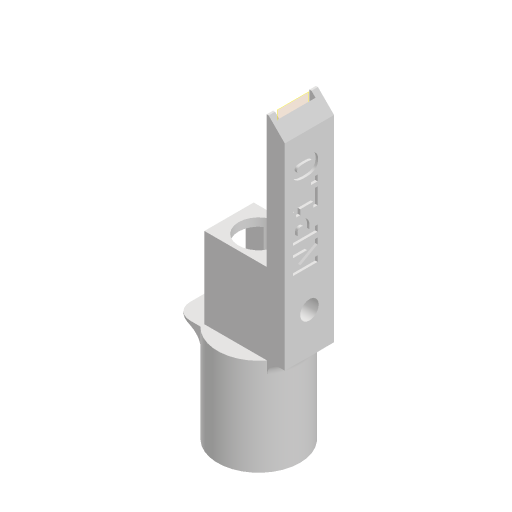
# Autodesk Inventor part: surgical_holder
Saved by Autodesk Inventor 2023 (Build 270158000, 158)
## iProperties
Created: 2023-01-31
Part Number: surgical_holder
Material: Generic
Document SubType Name: Modeling
Designer: mmelin
Density: 1 g/cm^3
Appearance: Default
Author: mmelin
Autodesk Inventor part; units mm, degrees
ref_plane "YZ Plane" through (0, 0, 0) normal (1, 0, 0) x (0, 1, 0)
ref_plane "XZ Plane" through (0, 0, 0) normal (0, 1, 0) x (-1, 0, 0)
ref_plane "XY Plane" through (0, 0, 0) normal (0, 0, 1) x (1, 0, 0)
ref_plane "Work Plane2" through (0.5918, -11.5934, -3.2844) normal (1, 0, 0) x (0, 0, -1)
sketch "Sketch2" plane through (0.5918, -11.5934, -3.2844) normal (1, 0, 0) x (0, 0, -1)
  line L0 (0.8156, 0) -> (0.8156, -11.35) projected
  line L1 (-3.2844, 0) -> (-3.2844, -15.35) projected
  line L2 (0.8156, 0) -> (-3.2844, 0) projected
  line L3 (1.8156, 0) -> (-4.2844, 0)
  line L4 (-4.2844, 0) -> (-4.2844, -11.35)
  line L5 (-4.2844, -11.35) -> (1.8156, -11.35)
  line L6 (1.8156, -11.35) -> (1.8156, 0)
  line L7 (0.8156, -11.35) -> (-2.0046, -11.35) projected
  point P0 (-3.2844, 11.5934)
  point P1 (0.8156, 0)
  point P2 (0.8156, -11.35)
  point P3 (-3.2844, -11.35)
  dimension "d81" = 1
  dimension "d82" = 1
  constraints: 8 end point, 2 collinear, 2 parallel, 1 horizontal, 1 perpendicular
  measures "d81" distance between parallel lines of L6 L0
  measures "d82" distance between parallel lines of L1 L4
extrude "arm_base" add sketch "Sketch2" along normal blind 1.5
sketch "Sketch22" plane through (0.5918, -11.5934, -3.2844) normal (-1, 0, 0) x (0, 0, 1)
  line L0 (4.2844, -11.35) -> (-1.8156, -11.35) projected
  line L1 (-1.8156, -11.35) -> (-1.0156, -11.35)
  line L2 (-1.0156, -11.35) -> (-1.0156, 0)
  line L3 (-1.0156, 0) -> (-1.8156, 0)
  line L4 (-1.8156, 0) -> (-1.8156, -11.35)
  line L5 (4.2844, -11.35) -> (-1.8156, -11.35) projected
  line L6 (4.2844, -11.35) -> (3.4844, -11.35)
  line L7 (3.4844, -11.35) -> (3.4844, 0)
  line L8 (3.4844, 0) -> (4.2844, 0)
  line L9 (4.2844, 0) -> (4.2844, -11.35)
  line L10 (-0.8156, 0) -> (-0.8156, -11.35) projected
  line L11 (3.2844, 0) -> (3.2844, -15.35) projected
  line L12 (-1.8156, 0) -> (4.2844, 0) projected
  point P0 (3.2844, 11.5934)
  point P1 (3.4844, -11.35)
  dimension "d83" = 0.2
  dimension "d84" = 0.2
  constraints: 16 end point, 4 parallel, 2 horizontal, 2 perpendicular, 1 collinear, 1 point on line
  measures "d83" distance between parallel lines of L10 L2
  measures "d84" distance between parallel lines of L11 L7
extrude "arm_tabs" add sketch "Sketch22" along normal blind 0.75 contours L0 L7 L8 L9 | L0 L4 L3 L2
sketch "Sketch23" plane through (2.0918, -22.9434, -5.1) normal (0, -1, 0) x (1, 0, 0)
  line L0 (-1.5, 0.8) -> (-2.25, 0.8) projected
  line L1 (-2.25, 0) -> (-2.25, 0.8) projected
  line L2 (-2.25, 5.3) -> (-2.25, 6.1) projected
  line L3 (-1.5, 5.3) -> (-2.25, 5.3) projected
  line L4 (-1.5, 5.3) -> (-1.5, 0.8) projected
  line L5 (0, 6.1) -> (0, 0) projected
  line L6 (-2.25, 6.1) -> (0, 6.1) projected
  line L7 (-1.5, 0.8) -> (-2.008, 0.8)
  line L8 (-2.008, 0.8) -> (-2.008, 3.8182)
  line L9 (-2.008, 3.8182) -> (-1.5, 3.8182)
  line L10 (-1.5, 3.8182) -> (-1.5, 0.8)
  line L11 (-2.25, 0) -> (0, 0) projected
  line L12 (-1.5, 0.8) -> (-2.25, 0.8) projected
  line L13 (-2.25, 0) -> (-2.25, 0.8) projected
  line L14 (-2.25, 5.3) -> (-2.25, 6.1) projected
  line L15 (-1.5, 5.3) -> (-2.25, 5.3) projected
  line L16 (-2.25, 0) -> (0, 0) projected
  line L17 (-2.008, 0.9187) -> (-2.008, 4.0182)
  line L18 (-2.9625, 4.0182) -> (-1.5, 4.0182) projected
  point P0 (-2.0918, 5.1)
  point P1 (0, 0)
  point P2 (-1.5, 5.2)
  point P3 (-1.5, 0.9)
  point P4 (-1.5, 3.8182)
  point P5 (0, 6.1)
  point P6 (-2.25, 6.1)
  dimension "d145" = 0.508
  dimension "d146" = 0.2
  constraints: 10 end point, 2 parallel, 2 perpendicular, 1 collinear, 1 horizontal, 1 point on line, 3 other
  measures "d145" distance between parallel lines of L17 L4
  measures "d146" distance between parallel lines of L18 L9
extrude "cut_out" add sketch "Sketch23" along normal blind 15 contours L4 L3 L2 L6 L5 L11 L1 L0 | L0 L8 L9 L4
chamfer "Chamfer1" distance 2 angle 45 1 edges at (2.0918, -11.5934, -2.05)
sketch "Sketch25" plane through (-0.1582, -11.5934, -3.2844) normal (-1, 0, 0) x (0, 0, 1)
  line L0 (0.0652, -16.35) -> (3.0834, -16.35)
  line L1 (4.2844, -26.35) -> (4.2844, -16.35)
  line L2 (4.2844, -16.35) -> (-1.8156, -16.35)
  line L3 (-1.8156, -16.35) -> (-1.8156, -26.35)
  line L4 (-1.8156, 0) -> (-1.8156, -26.35) projected
  line L5 (4.2844, 0) -> (4.2844, -26.35) projected
  line L6 (-1.8156, -26.35) -> (4.2844, -26.35)
  line L7 (4.2844, -26.35) -> (3.4844, -26.35) projected
  point P0 (3.2844, 11.5934)
  dimension "d131" = 10
  constraints: 10 end point, 4 collinear, 1 parallel
  measures "d131" distance between parallel lines of L2 L6
extrude "slider_box" add sketch "Sketch25" along normal blind 7.7
sketch "Sketch26" plane through (-7.8582, -11.5934, -3.2844) normal (-1, 0, 0) x (0, 0, 1)
  line L0 (-1.8156, -26.35) -> (4.2844, -26.35) projected
  line L1 (3.2844, -25.35) -> (-0.8156, -25.35)
  line L2 (-0.8156, -25.35) -> (-0.8156, -17.35)
  line L3 (-0.8156, -17.35) -> (3.2844, -17.35)
  line L4 (3.2844, -17.35) -> (3.2844, -25.35)
  line L5 (4.2844, -26.35) -> (4.2844, -16.35) projected
  line L6 (4.2844, -16.35) -> (-1.8156, -16.35) projected
  line L7 (-1.8156, -16.35) -> (-1.8156, -26.35) projected
  point P0 (3.2844, 11.5934)
  dimension "d97" = 1
  dimension "d147" = 1
  dimension "d148" = 1
  dimension "d149" = 1
  constraints: 8 end point, 2 parallel, 1 horizontal, 1 perpendicular
  measures "d97" distance between parallel lines of L0 L1
  measures "d147" distance between parallel lines of L5 L4
  measures "d148" distance between parallel lines of L6 L3
  measures "d149" distance between parallel lines of L7 L2
extrude "slider_cutout" cut sketch "Sketch26" against normal blind 7.7 contours L1 L2 L3 L4
sketch "Sketch27" plane through (2.0918, -37.9434, -5.1) normal (0, -1, 0) x (1, 0, 0)
  circle A0 centre (-6.2786, 3.05) radius 5.1
  line L0 (0.1377, 6.1) -> (-9.3123, 6.1)
  line L1 (0, 0) -> (-9.95, 0) projected
  line L2 (-6.2786, 3.05) -> (-6.2786, 0) construction
  line L3 (-6.2786, 3.05) -> (-6.2786, 6.1) construction
  line L4 (-11.0572, 5.1) -> (-11.0572, 1) projected
  line L5 (-1.5, 1) -> (-1.5, 5.1) projected
  line L6 (-6.2786, 3.05) -> (-11.0572, 3.05) construction
  line L7 (-6.2786, 3.05) -> (-1.5, 3.05) construction
  line L8 (0, 6.1) -> (-9.95, 6.1) projected
  point P0 (-2.0918, 5.1)
  point P1 (-9.95, 0)
  point P2 (-2.25, 0.019)
  dimension "d103" = 10.2
  constraints: 10 end point, 3 collinear, 2 midpoint, 2 point on line, 1 centre point, 1 vertical, 2 other
  measures "d103" diameter of A0
extrude "cylinder_post" add sketch "Sketch27" along normal blind 12
fillet "Fillet2" radius 1.8 1 edges at (-3.9788, -37.9434, -5.1)
sketch "Sketch28" plane through (-4.1868, -49.9434, -2.05) normal (0, -1, 0) x (1, 0, 0)
  circle A0 centre (0, 0) radius 5.1 projected
  circle A1 centre (0, 0) radius 4.1
  point P0 (4.1868, 2.05)
  dimension "d108" = 8.2
  constraints: 1 centre point, 1 coincident
  measures "d108" diameter of A1
extrude "post_cutout" cut sketch "Sketch28" against normal blind 9 contours A1
sketch "Sketch29" plane through (-4.1868, -40.9434, -2.05) normal (0, -1, 0) x (1, 0, 0)
  circle A0 centre (0, 0) radius 4.1 projected
  circle A1 centre (0, 0) radius 2.9
  point P0 (4.1868, 2.05)
  dimension "d111" = 5.8
  constraints: 1 centre point, 1 coincident
  measures "d111" diameter of A1
extrude "well" add sketch "Sketch29" along normal blind 8
fillet "Fillet4" radius 2 1 edges at (-0.0993, -37.0434, -5.1)
sketch "Sketch32" plane through (2.0918, -11.5934, -3.2844) normal (1, 0, 0) x (0, 0, -1)
  circle A0 centre (-1.2344, -21.35) radius 1.15
  line L0 (-1.2344, -21.35) -> (-1.2344, -25.35) construction
  line L1 (-1.2344, -21.35) -> (-1.2344, -17.35) construction
  line L2 (-1.2344, -21.35) -> (-3.2844, -21.35) construction
  line L3 (-1.2344, -21.35) -> (0.8156, -21.35) construction
  line L4 (-3.2844, -17.35) -> (-3.2844, -25.35) projected
  line L5 (0.8156, -17.35) -> (-3.2844, -17.35) projected
  line L6 (-3.2844, -25.35) -> (0.8156, -25.35) projected
  line L7 (0.8156, -25.35) -> (0.8156, -17.35) projected
  point P0 (-3.2844, 11.5934)
  dimension "d122" = 2.3
  constraints: 8 end point, 4 midpoint, 3 collinear, 2 perpendicular, 1 centre point, 1 point on line, 1 vertical
  measures "d122" diameter of A0
sketch "Sketch33" plane through (2.0918, -37.9434, -5.1) normal (0, 1, 0) x (1, 0, 0)
  arc A0 (-9.95, 0.4899) -> (-2.1911, -6.1) centre (-6.2786, -3.05) ccw projected
  line L0 (-9.95, -6.5899) -> (-13.23, -6.5899)
  line L1 (-13.23, -6.5899) -> (-13.23, 0.4899)
  line L2 (-13.23, 0.4899) -> (-9.95, 0.4899)
  line L3 (-9.95, 0.4899) -> (-9.95, -6.5899)
  point P0 (-2.0918, -5.1)
  point P1 (-1.6215, -0.9)
  point P2 (-1.5, -4.8319)
  point P3 (-9.4673, -7.0302)
  point P4 (-9.45, 0.918)
  point P5 (-9.45, -7.044)
  point P6 (-9.45, 0.918)
  dimension "d137" = 3.28
  constraints: 8 end point, 2 parallel, 1 horizontal, 1 perpendicular, 1 point on circle
  measures "d137" distance of L0.start L0.end
extrude "side_tab" add sketch "Sketch33" against normal blind 0.2
fillet "Fillet5" radius 2 1 edges at (-9.2868, -38.1434, -2.05)
fillet "Fillet6" radius 2 2 edges at (-11.1382, -38.0434, 1.4899) (-11.1382, -38.0434, -5.5899)
sketch "Sketch36" plane through (-0.1582, -27.9434, 0.2) normal (0, 1, 0) x (1, 0, 0)
  line L0 (0.75, 1.4818) -> (0.242, 1.4818) projected
  line L1 (0.242, 1.4818) -> (0.75, 1.4818)
  line L2 (0.75, 1.4818) -> (0.75, 0)
  line L3 (0.75, 0) -> (0.242, 0)
  line L4 (0.242, 0) -> (0.242, 1.4818)
  line L5 (0, 0) -> (0, 4.5) projected
  line L6 (0.242, 1.4818) -> (0.242, 4.5) projected
  line L7 (0, 4.5) -> (0.242, 4.5)
  line L8 (0, 0) -> (0, -0.8) projected
  line L9 (0, 0) -> (0.242, 0)
  point P0 (0.1582, 0.2)
  point P1 (0.75, 1.4818)
  point P2 (0, -0.9)
  constraints: 12 end point, 2 parallel, 2 perpendicular, 1 horizontal
extrude "fill_gaps" add sketch "Sketch36" against normal up to surface (10 mm away)
extrude "screw_hole" cut sketch "Sketch32" against normal up to surface (2.25 mm away) contours A0
fillet "Fillet7" radius 1.5 2 edges at (0.6535, -37.9434, -0.4432) (0.5192, -37.9434, -4.0156)
sketch "Sketch37" plane through (-4.1868, -40.9434, -2.05) normal (0, -1, 0) x (1, 0, 0)
  circle A0 centre (0, 0) radius 4.1 projected
  circle A1 centre (0, 0) radius 1.5
  point P0 (4.1868, 2.05)
  dimension "d138" = 3
  constraints: 1 centre point, 1 coincident
  measures "d138" diameter of A1
extrude "screw_hole_2" cut sketch "Sketch37" against normal up to surface (13 mm away) contours A1
sketch "Sketch38" plane through (-0.1582, -27.9434, 1) normal (0, 1, 0) x (-1, 0, 0)
  circle A0 centre (4.0286, -3.05) radius 1.5 projected
  circle A1 centre (4.0286, -3.05) radius 2.5
  point P0 (-0.1582, -1)
  dimension "d141" = 5
  constraints: 1 centre point, 1 coincident
  measures "d141" diameter of A1
extrude "screw_hole_3" cut sketch "Sketch38" against normal blind 11
sketch "Sketch39" plane through (2.0918, -11.5934, -3.2844) normal (1, 0, 0) x (0, 0, -1)
  line L0 (-3.3432, -17.034) -> (-3.3432, -3.22) construction
  line L1 (-3.3432, -3.22) -> (1.1831, -3.22) construction
  line L2 (1.1831, -3.22) -> (1.1831, -17.034) construction
  line L3 (1.1831, -17.034) -> (-3.3432, -17.034) construction
  line L4 (-0.2314, -14.1052) -> (-0.2314, -14.8417)
  line L5 (-0.2314, -14.8417) -> (-2.357, -16.0182)
  line L6 (-2.357, -16.0182) -> (-0.2314, -16.0182)
  line L7 (-0.2314, -16.0182) -> (-0.2314, -16.7177)
  line L8 (-0.2314, -16.7177) -> (-3.2814, -16.7177)
  line L9 (-3.2814, -16.7177) -> (-3.2814, -15.7785)
  line L10 (-3.2814, -15.7785) -> (-1.5339, -14.8046)
  line L11 (-1.5339, -14.8046) -> (-3.2814, -14.8046)
  line L12 (-3.2814, -14.8046) -> (-3.2814, -14.1052)
  line L13 (-3.2814, -14.1052) -> (-0.2314, -14.1052)
  spline S0 degree 2 poles (-2.3199, -11.1392) (-2.1074, -11.1392) (-1.7218, -11.2751) (-1.5933, -11.4012) knots 0 0 0 1 2 2 2
  spline S1 degree 2 poles (-1.5933, -11.4012) (-1.5117, -11.4778) (-1.3782, -11.6657) (-1.3313, -11.7769) knots 0 0 0 1 2 2 2
  spline S2 degree 2 poles (-1.3313, -11.7769) (-1.2843, -11.8906) (-1.2299, -12.155) (-1.2299, -12.3182) knots 0 0 0 1 2 2 2
  line L14 (-1.2299, -12.3182) -> (-1.2299, -12.7186)
  line L15 (-1.2299, -12.7186) -> (-0.2314, -12.7186)
  line L16 (-0.2314, -12.7186) -> (-0.2314, -13.4848)
  line L17 (-0.2314, -13.4848) -> (-3.2814, -13.4848)
  line L18 (-3.2814, -13.4848) -> (-3.2814, -12.3009)
  spline S3 degree 2 poles (-3.2814, -12.3009) (-3.2814, -12.0389) (-3.185, -11.6558) (-3.0812, -11.5001) knots 0 0 0 1 2 2 2
  spline S4 degree 2 poles (-3.0812, -11.5001) (-2.965, -11.327) (-2.5844, -11.1392) (-2.3199, -11.1392) knots 0 0 0 1 2 2 2
  spline S5 degree 2 poles (-2.3001, -11.9252) (-2.4311, -11.9252) (-2.6165, -12.0488) (-2.6511, -12.1328) knots 0 0 0 1 2 2 2
  spline S6 degree 2 poles (-2.6511, -12.1328) (-2.6981, -12.2415) (-2.7129, -12.4393) (-2.7129, -12.6098) knots 0 0 0 1 2 2 2
  line L19 (-2.7129, -12.6098) -> (-2.7129, -12.7186)
  line L20 (-2.7129, -12.7186) -> (-1.7984, -12.7186)
  line L21 (-1.7984, -12.7186) -> (-1.7984, -12.6642)
  spline S7 degree 2 poles (-1.7984, -12.6642) (-1.7984, -12.5579) (-1.8033, -12.3651) (-1.8157, -12.2935) knots 0 0 0 1 2 2 2
  spline S8 degree 2 poles (-1.8157, -12.2935) (-1.8256, -12.2317) (-1.8849, -12.0957) (-1.922, -12.0586) knots 0 0 0 1 2 2 2
  spline S9 degree 2 poles (-1.922, -12.0586) (-1.9961, -11.9796) (-2.1617, -11.9252) (-2.3001, -11.9252) knots 0 0 0 1 2 2 2
  line L22 (-0.2314, -8.6305) -> (-0.2314, -10.6449)
  line L23 (-0.2314, -10.6449) -> (-0.7628, -10.6449)
  line L24 (-0.7628, -10.6449) -> (-0.7628, -10.0022)
  line L25 (-0.7628, -10.0022) -> (-2.3768, -10.0022)
  line L26 (-2.3768, -10.0022) -> (-2.3768, -10.6449)
  line L27 (-2.3768, -10.6449) -> (-2.8736, -10.6449)
  spline S10 degree 2 poles (-2.8736, -10.6449) (-2.8736, -10.504) (-2.9106, -10.2247) (-2.9502, -10.1407) knots 0 0 0 1 2 2 2
  spline S11 degree 2 poles (-2.9502, -10.1407) (-2.9996, -10.0443) (-3.1652, -9.9355) (-3.2888, -9.9256) knots 0 0 0 1 2 2 2
  line L28 (-3.2888, -9.9256) -> (-3.2888, -9.2583)
  line L29 (-3.2888, -9.2583) -> (-0.7628, -9.2583)
  line L30 (-0.7628, -9.2583) -> (-0.7628, -8.6305)
  line L31 (-0.7628, -8.6305) -> (-0.2314, -8.6305)
  line L32 (-0.2314, -7.3576) -> (-0.2314, -8.0818)
  line L33 (-0.2314, -8.0818) -> (-1.0371, -8.0818)
  line L34 (-1.0371, -8.0818) -> (-1.0371, -7.3576)
  line L35 (-1.0371, -7.3576) -> (-0.2314, -7.3576)
  spline S12 degree 2 poles (-1.7564, -4.5523) (-1.3609, -4.5523) (-0.7677, -4.6783) (-0.5675, -4.8192) knots 0 0 0 1 2 2 2
  spline S13 degree 2 poles (-0.5675, -4.8192) (-0.3698, -4.9576) (-0.1671, -5.405) (-0.1671, -5.7263) knots 0 0 0 1 2 2 2
  spline S14 degree 2 poles (-0.1671, -5.7263) (-0.1671, -6.0501) (-0.3698, -6.495) (-0.5725, -6.6359) knots 0 0 0 1 2 2 2
  spline S15 degree 2 poles (-0.5725, -6.6359) (-0.7727, -6.7768) (-1.3609, -6.9028) (-1.7564, -6.9028) knots 0 0 0 1 2 2 2
  spline S16 degree 2 poles (-1.7564, -6.9028) (-2.1617, -6.9028) (-2.7352, -6.7768) (-2.9428, -6.6334) knots 0 0 0 1 2 2 2
  spline S17 degree 2 poles (-2.9428, -6.6334) (-3.1454, -6.49) (-3.3432, -6.0377) (-3.3432, -5.7263) knots 0 0 0 1 2 2 2
  spline S18 degree 2 poles (-3.3432, -5.7263) (-3.3432, -5.3976) (-3.1356, -4.9576) (-2.9304, -4.8167) knots 0 0 0 1 2 2 2
  spline S19 degree 2 poles (-2.9304, -4.8167) (-2.7302, -4.6783) (-2.1395, -4.5523) (-1.7564, -4.5523) knots 0 0 0 1 2 2 2
  spline S20 degree 2 poles (-1.7564, -5.321) (-2.3224, -5.321) (-2.7796, -5.5063) (-2.7796, -5.7263) knots 0 0 0 1 2 2 2
  spline S21 degree 2 poles (-2.7796, -5.7263) (-2.7796, -5.9463) (-2.3224, -6.1341) (-1.7539, -6.1341) knots 0 0 0 1 2 2 2
  spline S22 degree 2 poles (-1.7539, -6.1341) (-1.1953, -6.1341) (-0.7307, -5.9463) (-0.7307, -5.7263) knots 0 0 0 1 2 2 2
  spline S23 degree 2 poles (-0.7307, -5.7263) (-0.7307, -5.5088) (-1.1953, -5.321) (-1.7564, -5.321) knots 0 0 0 1 2 2 2
  point P0 (-3.2844, 11.5934)
  constraints: 2 other
emboss "Emboss1" sketch "Sketch39" operation cut depth 0.3 direction (-1, 0, 0)
equation "\"d84\" = d83"
body "Solid1"
